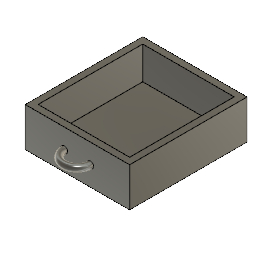
Gavetas v3 (Autodesk Fusion 360 design; units mm, degrees)
Autodesk Fusion 360 part; units mm, degrees
sketch "Sketch1" plane through (0, 0, 0) normal (0, 1, 0) x (1, 0, 0)
  line L0 (40, 15) -> (-40, 15)
  line L1 (-40, 15) -> (-40, -15)
  line L2 (-40, -15) -> (40, -15)
  line L3 (40, -15) -> (40, 15)
  line L4 (40, 15) -> (-40, -15) construction
  line L5 (-40, 15) -> (40, -15) construction
  dimension "d1" = 80
  dimension "d2" = 30
  constraint horizontal L0
  constraint perpendicular L0 L1
  constraint parallel L0 L2
  constraint parallel L1 L3
  constraint coincident L4 origin
  constraint coincident L5 origin
  measures "d1" distance of L1.end L2.end
  measures "d2" distance of L0.end L1.end
extrude "Extrude1" add sketch "Sketch1" along normal blind 90
shell "Shell1" thickness 5 removed faces 1 at (-13.3333, 60, 15)
ref_plane "WorkPlane1" through (0, 45, -15) normal (0, 0, 1) x (1, 0, 0)
sketch "Sketch2" plane through (0, 45, -15) normal (0, 0, 1) x (1, 0, 0)
  arc A0 (-10, -45) -> (10, -45) centre (0, -45) ccw
pipe "Pipe1" add diameter 5 wall 1.25 path "Sketch2" along A0
move_face "MoveFace1" to x (1, 0, 0) y (0, 1, 0) z (0, 0, 1) at (0, 0, 15) 1 faces at (-9.4601, -7.9379, -14.1449)
